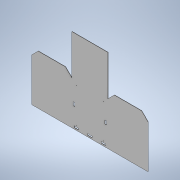
# Autodesk Inventor part: head_without_face
Saved by Autodesk Inventor 2021.1 (Build 251245010, 245A)
## iProperties
Created: 2023-01-11
Part Number: head_without_face
Material: Типовые
Document SubType Name: Modeling
Designer: zmoze
Density: 1 g/cm^3
Appearance: По умолчанию
Author: zmoze
Autodesk Inventor part; units mm, degrees
ref_plane "YZ Plane" through (0, 0, 0) normal (1, 0, 0) x (0, 1, 0)
ref_plane "XZ Plane" through (0, 0, 0) normal (0, 1, 0) x (-1, 0, 0)
ref_plane "XY Plane" through (0, 0, 0) normal (0, 0, 1) x (1, 0, 0)
sketch "Эскиз1" plane through (0, 0, 0) normal (0, 0, 1) x (1, 0, 0)
  line L0 (0, 0) -> (810, 0)
  line L1 (810, 0) -> (810, 300)
  line L2 (810, 300) -> (0, 300)
  line L3 (0, 300) -> (0, 0)
  line L4 (280, 300) -> (530, 300) construction
  line L5 (530, 300) -> (530, 0) construction
  line L6 (530, 0) -> (280, 0) construction
  line L7 (280, 0) -> (280, 300) construction
  line L8 (280, 300) -> (530, 300)
  line L9 (530, 300) -> (530, 580)
  line L10 (530, 580) -> (280, 580)
  line L11 (280, 580) -> (280, 300)
  line L12 (0, 300) -> (45, 345)
  line L13 (45, 345) -> (235, 345)
  line L14 (235, 345) -> (280, 300)
  line L15 (530, 300) -> (575, 345)
  line L16 (575, 345) -> (765, 345)
  line L17 (765, 345) -> (810, 300)
  dimension "d0" = 300
  dimension "d1" = 810
  dimension "d2" = 250
  dimension "d3" = 280
  dimension "d4" = 280
  dimension "d5" = 280
  dimension "d6" = 45
  constraints: 36 end point, 7 perpendicular, 6 parallel, 4 horizontal, 4 point on line
  measures "d0" distance of L2.end L0.start
  measures "d1" distance of L0.start L0.end
  measures "d2" distance between parallel lines of L5 L7
  measures "d3" distance between parallel lines of L1 L5
  measures "d4" distance of L8.end L9.end
  measures "d5" distance between parallel lines of L1 L9
  measures "d6" distance between parallel lines of L2 L16
extrude "Выдавливание1" add sketch "Эскиз1" along normal blind 2
sketch "Эскиз2" plane through (0, 0, 2) normal (0, 0, 1) x (1, 0, 0)
  line L0 (45, 345) -> (0, 300) projected
  line L1 (0, 300) -> (0, 0) projected
  line L2 (0, 0) -> (810, 0) projected
  line L3 (810, 0) -> (810, 300) projected
  line L4 (810, 300) -> (765, 345) projected
  line L5 (765, 345) -> (575, 345) projected
  line L6 (575, 345) -> (530, 300) projected
  line L7 (530, 300) -> (530, 580) projected
  line L8 (530, 580) -> (280, 580) projected
  line L9 (280, 580) -> (280, 300) projected
  line L10 (280, 300) -> (235, 345) projected
  line L11 (235, 345) -> (45, 345) projected
  line L12 (280, 300) -> (530, 300) construction
  line L13 (530, 300) -> (530, 0) construction
  line L14 (530, 0) -> (280, 0) construction
  line L15 (280, 0) -> (280, 300) construction
  line L16 (530, 300) -> (530, 580) construction
  circle A0 centre (310, 270) radius 1.5
  circle A1 centre (500, 270) radius 1.5
  circle A2 centre (310, 30) radius 1.5
  circle A3 centre (500, 30) radius 1.5
  line L17 (500, 270) -> (310, 270) construction
  line L18 (310, 270) -> (310, 30) construction
  line L19 (310, 30) -> (500, 30) construction
  line L20 (500, 30) -> (500, 270) construction
  line L21 (290, 162.5) -> (300, 162.5)
  line L22 (300, 162.5) -> (300, 137.5)
  line L23 (300, 137.5) -> (290, 137.5)
  line L24 (290, 137.5) -> (290, 162.5)
  line L25 (510, 162.5) -> (520, 162.5)
  line L26 (520, 162.5) -> (520, 137.5)
  line L27 (520, 137.5) -> (510, 137.5)
  line L28 (510, 137.5) -> (510, 162.5)
  line L29 (280, 150) -> (530, 150) construction
  line L30 (390, 20) -> (420, 20)
  line L31 (420, 20) -> (420, 10)
  line L32 (420, 10) -> (390, 10)
  line L33 (390, 10) -> (390, 20)
  line L34 (405, 300) -> (405, 0) construction
  line L35 (0, 0) -> (810, 0) construction
  line L36 (325, 10) -> (295, 10)
  line L37 (295, 10) -> (295, 20)
  line L38 (295, 20) -> (325, 20)
  line L39 (325, 20) -> (325, 10)
  line L40 (485, 10) -> (515, 10)
  line L41 (515, 10) -> (515, 20)
  line L42 (515, 20) -> (485, 20)
  line L43 (485, 20) -> (485, 10)
  point P0 (290, 150)
  point P1 (510, 150)
  point P2 (405, 20)
  dimension "d9" = 3
  dimension "d10" = 30
  dimension "d11" = 30
  dimension "d12" = 30
  dimension "d13" = 30
  dimension "d16" = 10
  dimension "d17" = 25
  dimension "d18" = 10
  dimension "d19" = 10
  dimension "d20" = 10
  dimension "d21" = 30
  dimension "d22" = 10
  dimension "d23" = 30
  dimension "d24" = 15
  constraints: 60 end point, 10 parallel, 7 horizontal, 7 midpoint, 5 perpendicular, 4 centre point, 4 point on line, 4 symmetric about line, 3 collinear, 3 equal radius, 2 equal length, 2 vertical
  measures "d9" diameter of A0
  measures "d10" distance from line of L12 L17.end
  measures "d11" distance from line of L15 L17.end
  measures "d12" distance between parallel lines of L14 L19
  measures "d13" distance between parallel lines of L13 L20
  measures "d16" distance of L21.start L21.end
  measures "d17" distance of L21.end L22.end
  measures "d18" distance between parallel lines of L15 L24
  measures "d19" distance between parallel lines of L13 L26
  measures "d20" distance of L30.end L31.end
  measures "d21" distance of L30.start L30.end
  measures "d22" distance between parallel lines of L35 L32
  measures "d23" distance of L36.start L36.end
  measures "d24" distance between parallel lines of L15 L37
extrude "Выдавливание2" cut sketch "Эскиз2" against normal through all contours A0 | A1 | A2 | A3 | L21 L22 L23 L24 | L25 L26 L27 L28 | L30 L31 L32 L33 | L36 L37 L38 L39 | L43 L42 L41 L40
